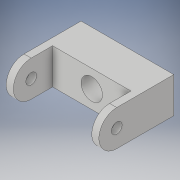
# Autodesk Inventor part: Muñeca
Saved by Autodesk Inventor 2019 (Build 230136000, 136)
## iProperties
Created: 2019-10-18
Part Number: Muñeca
Material: Genérico
Document SubType Name: Modeling
Designer: Josue
Density: 1 g/cm^3
Appearance: Valor por defecto
Author: Josue
Autodesk Inventor part; units mm, degrees
ref_plane "YZ Plane" through (0, 0, 0) normal (1, 0, 0) x (0, 1, 0)
ref_plane "XZ Plane" through (0, 0, 0) normal (0, 1, 0) x (-1, 0, 0)
ref_plane "XY Plane" through (0, 0, 0) normal (0, 0, 1) x (1, 0, 0)
sketch "Boceto1" plane through (0, 0, 0) normal (0, 0, 1) x (1, 0, 0)
  line L0 (65, -25) -> (-65, -25)
  line L1 (-65, -25) -> (-65, 25)
  line L2 (-65, 25) -> (65, 25)
  line L3 (65, 25) -> (65, -25)
  line L4 (65, -25) -> (-65, 25) construction
  line L5 (-65, -25) -> (65, 25) construction
  point P0 (0, 0)
  dimension "d0" = 130
  dimension "d1" = 50
  constraints: 12 end point, 2 midpoint, 2 parallel, 1 horizontal, 1 perpendicular
  measures "d0" distance of L1.end L2.end
  measures "d1" distance of L0.end L1.end
extrude "Extrusión1" add sketch "Boceto1" along normal blind 50
sketch "Boceto2" plane through (65, -25, 0) normal (1, 0, 0) x (0, 0, -1)
  line L0 (-50, 0) -> (-80, 0)
  line L1 (-50, 0) -> (-50, 50) projected
  line L2 (-50, 50) -> (-80, 50)
  arc A0 (-80, 50) -> (-80, 0) centre (-80, 25) ccw
  circle A1 centre (-80, 25) radius 7.5
  point P0 (0, 25)
  dimension "d4" = 30
  dimension "d5" = 30
  dimension "d6" = 15
  constraints: 4 end point, 2 centre point, 2 horizontal, 2 point on circle, 1 coincident, 1 tangent
  measures "d4" distance of L0.start L0.end
  measures "d5" distance of L1.end L2.end
  measures "d6" diameter of A1
extrude "Extrusión2" add sketch "Boceto2" against normal blind 10
sketch "Boceto3" plane through (-65, -25, 0) normal (-1, 0, 0) x (0, 0, 1)
  circle A0 centre (80, 25) radius 7.5 projected
  arc A1 (80, 0) -> (80, 50) centre (80, 25) ccw projected
  line L0 (80, 50) -> (50, 50) projected
  line L1 (50, 50) -> (50, 0) projected
  line L2 (50, 0) -> (80, 0) projected
  point P0 (0, 25)
extrude "Extrusión3" add sketch "Boceto3" against normal blind 10
sketch "Boceto4" plane through (0, 0, 0) normal (0, 0, -1) x (-1, 0, 0)
  circle A0 centre (0, 0) radius 15
  dimension "d11" = 30
  constraints: 1 centre point, 1 coincident
  measures "d11" diameter of A0
extrude "Extrusión4" cut sketch "Boceto4" against normal up to next
